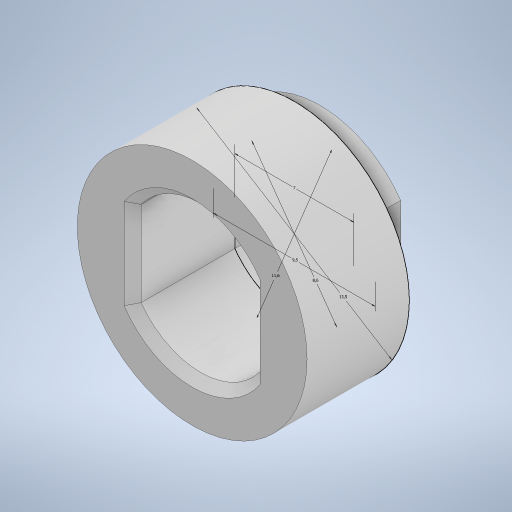
# Autodesk Inventor part: ANT_INSULATOR
Saved by Autodesk Inventor 2024 (Build 280153000, 153)
## iProperties
Created: 2026-02-20
Part Number: ANT_INSULATOR
Material: Типовые
Document SubType Name: Modeling
Designer: fm
Density: 1 g/cm^3
Appearance: По умолчанию
Author: fm
Autodesk Inventor part; units mm, degrees
ref_plane "YZ Plane" through (0, 0, 0) normal (1, 0, 0) x (0, 1, 0)
ref_plane "XZ Plane" through (0, 0, 0) normal (0, 1, 0) x (-1, 0, 0)
ref_plane "XY Plane" through (0, 0, 0) normal (0, 0, 1) x (1, 0, 0)
sketch "Эскиз1" plane through (0, 0, 0) normal (0, 0, 1) x (1, 0, 0)
  circle A0 centre (0, 0) radius 6.75
  circle A1 centre (0, 0) radius 5.8
  circle A2 centre (0, 0) radius 4.3
  line L0 (2.2504, 0) -> (3.5, 0)
  line L1 (3.5, 0) -> (-3.5, 0)
  line L2 (-3.5, -2.498) -> (-3.5, 2.498)
  line L3 (3.5, -2.498) -> (3.5, 2.498)
  line L4 (-4.75, 0) -> (4.75, 0)
  line L5 (-4.75, 3.3283) -> (-4.75, -3.3283)
  line L6 (4.75, -3.3283) -> (4.75, 3.3283)
  dimension "d0" = 13.5
  dimension "d1" = 11.6
  dimension "d2" = 8.6
  dimension "d3" = 7
  dimension "d4" = 9.5
  constraints: 14 end point, 6 midpoint, 4 coincident, 4 point on circle, 4 vertical, 3 centre point, 2 horizontal, 1 point on line
  measures "d0" diameter of A0
  measures "d1" diameter of A1
  measures "d2" diameter of A2
  measures "d3" distance of L1.end L0.end
  measures "d4" distance of L4.start L4.end
extrude "Выдавливание1" add sketch "Эскиз1" along normal blind 6 contours A0 | A1 L6 | L6 L4 A2 L5 A1 | A1 L5 L4 A2 L6 | L5 A1 | L4 L3 A2 | A2 L3 L4 | L4 L2 A2 | A2 L2 L4
extrude "Выдавливание2" add sketch "Эскиз1" against normal blind 1.5 contours L6 L4 A2 L5 A1 | A1 L5 L4 A2 L6 | L4 L3 A2 | A2 L3 L4 | L4 L2 A2 | A2 L2 L4
chamfer "Фаска1" distance 0.5 angle 45 4 edges at (0, 4.3, 6) (-3.5, 0, 6) (0, -4.3, 6) (3.5, 0, 6)
